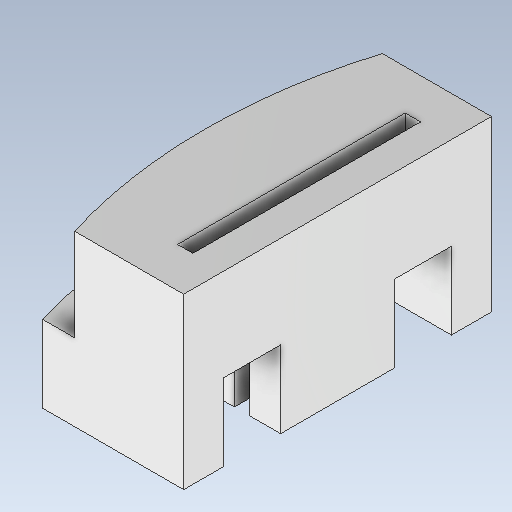
# Autodesk Inventor part: 555_CapAccessory_2
Saved by Autodesk Inventor 2021 (Build 250183000, 183)
## iProperties
Created: 2021-08-07
Part Number: 555_CapAccessory_2
Material: アセタール樹脂、白
Document SubType Name: Modeling
Designer: Hagihara Yuya
Density: 1.425 g/cm^3
Appearance: 滑らか - 白
Author: Hagihara Yuya
Autodesk Inventor part; units mm, degrees
ref_plane "YZ Plane" through (0, 0, 0) normal (1, 0, 0) x (0, 1, 0)
ref_plane "XZ Plane" through (0, 0, 0) normal (0, 1, 0) x (-1, 0, 0)
ref_plane "XY Plane" through (0, 0, 0) normal (0, 0, 1) x (1, 0, 0)
sketch "スケッチ1" plane through (0, 0, 0) normal (0, 0, 1) x (1, 0, 0)
  arc A0 (17.1875, -5) -> (17.1875, 5) centre (0, 0) ccw
  line L0 (17.9, -5) -> (12.6, -5)
  line L1 (12.6, -5) -> (12.6, 5)
  line L2 (12.6, 5) -> (17.9, 5)
  line L3 (17.9, 5) -> (17.9, -5)
  point P0 (12.6, 0)
  dimension "d0" = 17.9
  dimension "d1" = 10
  dimension "d2" = 5.3
  constraints: 8 end point, 2 parallel, 2 point on circle, 2 point on line, 1 centre point, 1 coincident, 1 horizontal, 1 horizontal alignment, 1 midpoint, 1 perpendicular, 1 tangent
  measures "d0" radius of A0
  measures "d1" distance of L0.end L1.end
  measures "d2" distance of L0.start L0.end
extrude "押し出し1" add sketch "スケッチ1" along normal blind 5.5 contours L0 L1 L2 A0
sketch "スケッチ2" plane through (0, 0, 0) normal (0, 0, -1) x (-1, 0, 0)
  line L0 (-12.6, 5) -> (-12.6, -5) projected
  line L1 (-12.6, -3.7) -> (-17.9, -3.7)
  line L2 (-17.9, -3.7) -> (-17.9, 3.7)
  line L3 (-17.9, 3.7) -> (-12.6, 3.7)
  line L4 (-12.6, 3.7) -> (-12.6, -3.7)
  line L5 (-12.6, 5) -> (-12.6, -5) projected
  line L6 (-12.6, -5) -> (-17.1875, -5) projected
  arc A0 (-17.1875, 5) -> (-17.1875, -5) centre (0, 0) ccw projected
  line L7 (-12.6, -1.85) -> (-17.9, -1.85)
  line L8 (-17.9, -1.85) -> (-17.9, 1.85)
  line L9 (-17.9, 1.85) -> (-12.6, 1.85)
  line L10 (-12.6, 1.85) -> (-12.6, -1.85)
  point P0 (-12.6, 0)
  point P1 (-12.6, 0)
  point P2 (-17.8041, -1.85)
  point P3 (-17.5134, -3.7)
  point P4 (-17.8041, 1.85)
  point P5 (-17.5134, 3.7)
  dimension "d5" = 1.3
  dimension "d6" = 3.7
  constraints: 16 end point, 4 midpoint, 4 parallel, 3 point on line, 2 horizontal, 2 perpendicular, 1 tangent
  measures "d5" distance between parallel lines of L6 L1
  measures "d6" distance between parallel lines of L9 L7
extrude "押し出し2" cut sketch "スケッチ2" against normal blind 2.5 contours L0 L9 A0 L3 | L0 L1 A0 L7
sketch "スケッチ3" plane through (0, 0, 0) normal (0, 0, -1) x (-1, 0, 0)
  line L0 (-12.6, -3.7) -> (-17.5134, -3.7) projected
  line L1 (-17.5134, 3.7) -> (-12.6, 3.7) projected
  line L2 (-13.6, -3.7) -> (-14.1, -3.7)
  line L3 (-14.1, -3.7) -> (-14.1, 3.7)
  line L4 (-14.1, 3.7) -> (-13.6, 3.7)
  line L5 (-13.6, 3.7) -> (-13.6, -3.7)
  line L6 (-12.6, 1.85) -> (-12.6, -1.85) projected
  point P0 (0, 0)
  dimension "d9" = 0.5
  dimension "d10" = 1
  constraints: 8 end point, 2 parallel, 2 point on line, 1 horizontal, 1 perpendicular
  measures "d9" distance between parallel lines of L3 L5
  measures "d10" distance between parallel lines of L6 L5
extrude "押し出し3" cut sketch "スケッチ3" against normal through all
sketch "スケッチ4" plane through (0, 0, 5.5) normal (0, 0, 1) x (1, 0, 0)
  line L0 (12.6, -5) -> (17.1875, -5) projected
  arc A0 (16.1434, -5) -> (16.1434, 5) centre (0, 0) ccw
  line L1 (17.1875, 5) -> (12.6, 5) projected
  arc A1 (17.1875, -5) -> (17.1875, 5) centre (0, 0) ccw projected
  dimension "d13" = 1
  constraints: 2 point on circle, 2 point on line, 1 centre point, 1 coincident
  measures "d13" radial gap between concentric circles of A1 A0
extrude "押し出し4" cut sketch "スケッチ4" against normal up to surface (3 mm away)
